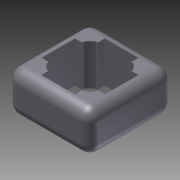
# Autodesk Inventor part: Frame_Support2
Saved by Autodesk Inventor 2011 SP2 (Build 150309200, 309)
## iProperties
Created: 2011-09-20
Part Number: Frame_Support2
Document SubType Name: Modeling
Designer: sungwook
Density: 8.08 g/cm^3
Material: Stainless Steel
Author: sungwook
Autodesk Inventor part; units mm, degrees
ref_plane "YZ Plane" through (0, 0, 0) normal (1, 0, 0) x (0, 1, 0)
ref_plane "XZ Plane" through (0, 0, 0) normal (0, 1, 0) x (-1, 0, 0)
ref_plane "XY Plane" through (0, 0, 0) normal (0, 0, 1) x (1, 0, 0)
sketch "Sketch1" plane through (0, 0, 0) normal (0, 0, 1) x (1, 0, 0)
  line L0 (-1.2075, 1.2085) -> (1.2075, 1.2085)
  line L1 (1.2075, 1.2085) -> (1.2075, -1.2085)
  line L2 (1.2075, -1.2085) -> (-1.2075, -1.2085)
  line L3 (-1.2075, -1.2085) -> (-1.2075, 1.2085)
  point P0 (0, 0)
  point P1 (0, 0)
  point P2 (0, 1.2085)
  point P3 (-1.2075, 0)
  dimension "d0" = 2.415
  dimension "d1" = 2.417
  constraints: 8 end point, 2 midpoint, 2 parallel, 1 horizontal, 1 horizontal alignment, 1 perpendicular, 1 vertical alignment
  measures "d0" distance of L0.start L0.end
  measures "d1" distance of L2.end L0.start
extrude "Extrusion1" add sketch "Sketch1" along normal blind 1.179
sketch "Sketch2" plane through (0, 0, 1.179) normal (0, 0, 1) x (1, 0, 0)
  line L0 (-0.705, 0.705) -> (-0.534, 0.705)
  line L1 (0.705, 0.705) -> (0.705, 0.534)
  line L2 (0.705, -0.705) -> (0.534, -0.705)
  line L3 (-0.705, -0.705) -> (-0.705, -0.534)
  line L4 (0, -1.6919) -> (0, 1.6919) projected
  line L5 (-1.6905, 0) -> (1.6905, 0) projected
  arc A0 (-0.534, 0.705) -> (-0.705, 0.534) centre (-0.3185, 0.3185) ccw
  arc A1 (0.705, 0.534) -> (0.534, 0.705) centre (0.3185, 0.3185) ccw
  arc A2 (-0.705, -0.534) -> (-0.534, -0.705) centre (-0.3185, -0.3185) ccw
  arc A3 (0.534, -0.705) -> (0.705, -0.534) centre (0.3185, -0.3185) ccw
  line L6 (0.705, -0.534) -> (0.705, -0.705)
  line L7 (0.534, -0.705) -> (-0.534, -0.705)
  line L8 (-0.534, -0.705) -> (-0.705, -0.705)
  line L9 (-0.705, -0.534) -> (-0.705, 0.534)
  line L10 (-0.705, 0.534) -> (-0.705, 0.705)
  line L11 (-0.534, 0.705) -> (0.534, 0.705)
  line L12 (0.534, 0.705) -> (0.705, 0.705)
  line L13 (0.705, 0.534) -> (0.705, -0.534)
  point P0 (0, 0)
  point P1 (-0.705, 0)
  point P2 (0, 0.705)
  dimension "d4" = 1.41
  dimension "d5" = 1.41
  dimension "d7" = 0.171
  dimension "d8" = 0.171
  constraints: 24 end point, 18 parallel, 9 perpendicular, 9 symmetric about line, 8 point on circle, 4 centre point, 3 horizontal, 1 horizontal alignment, 1 point on line, 1 vertical alignment, 3 other
  measures "d4" distance of L0.start L1.start
  measures "d5" distance of L1.start L2.start
  measures "d7" distance from line of L0.end L3
  measures "d8" distance from line of L0 L9.end
extrude "Extrusion2" cut sketch "Sketch2" against normal through all contours L11 L4 L5 L9 A0 | L11 A1 L13 L5 L4 | L5 L4 L7 A2 L9 | L5 L13 A3 L7 L4
sketch "Sketch3" plane through (0, 0, 1.179) normal (0, 0, 1) x (1, 0, 0)
  line L0 (-0.705, -0.534) -> (-0.705, 0.534) projected
  line L1 (-0.705, 0.485) -> (-0.915, 0.485)
  line L2 (-0.915, 0.485) -> (-0.915, -0.485)
  line L3 (-0.915, -0.485) -> (-0.705, -0.485)
  line L4 (-0.705, -0.485) -> (-0.705, 0.485)
  line L5 (-1.6905, 0) -> (1.6905, 0) projected
  line L6 (0, -1.6919) -> (0, 1.6919) projected
  point P0 (0, 0)
  point P1 (-0.915, 0)
  dimension "d11" = 0.21
  dimension "d12" = 0.97
  constraints: 8 end point, 2 parallel, 1 horizontal, 1 horizontal alignment, 1 midpoint, 1 perpendicular, 1 point on line
  measures "d11" distance of L1.start L1.end
  measures "d12" distance of L1.end L2.end
extrude "Extrusion3" cut sketch "Sketch3" against normal through all
pattern_circular "Circular Pattern1" count 4 over 360 about axis through (0, 0, -10) along (0, 0, 1) of "Extrusion3"
fillet "Fillet1" radius 0.31 12 edges at (-1.2075, 1.2085, 0.5895) (0, 1.2085, 1.179) (1.2075, 1.2085, 0.5895) (0, 1.2085, 0) (1.2075, 0, 0) (1.2075, 0, 1.179) (-1.2075, 0, 1.179) (-1.2075, 0, 0) (-1.2075, -1.2085, 0.5895) (0, -1.2085, 1.179) (0, -1.2085, 0) (1.2075, -1.2085, 0.5895)
body "Solid1"
